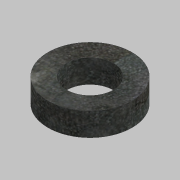
# Autodesk Inventor part: Two Piece Clamp Huco Stock No 046201030 Dim 30-54-15
Saved by Autodesk Inventor 2020.1 (Build 241239000, 239)
## iProperties
Created: 2019-08-27
Part Number: Two Piece Clamp Huco Stock No 046201030 Dim 30-54-15
Material: Steel
Document SubType Name: Modeling
Designer: Oliver Frolovs
Density: 7.85 g/cm^3
Appearance: Plate
Mass: 186.441 g
Surface Area: 71.2513 cm^2
Volume: 23.7504 cm^3
Huco30_54_15_TwoPieceClampWidth: 15.000 mm
Huco30_54_15_TwoPieceClampBore: 30.000 mm
Huco30_54_15_TwoPieceClampOuterDiameter: 54.000 mm
Author: Oliver Frolovs
Autodesk Inventor part; units mm, degrees
ref_plane "YZ Plane" through (0, 0, 0) normal (1, 0, 0) x (0, 1, 0)
ref_plane "XZ Plane" through (0, 0, 0) normal (0, 1, 0) x (-1, 0, 0)
ref_plane "XY Plane" through (0, 0, 0) normal (0, 0, 1) x (1, 0, 0)
sketch "Two Piece Clamp Profile" plane through (0, 0, 0) normal (0, 0, 1) x (1, 0, 0)
  circle A0 centre (0, 0) radius 15
  circle A1 centre (0, 0) radius 27
  dimension "d0" = 54
  dimension "d1" = 30
  constraints: 2 centre point, 2 coincident
  measures "d0" diameter of A1
  measures "d1" diameter of A0
extrude "Make Clamp by Extrusion" add sketch "Two Piece Clamp Profile" along normal mid plane 15
equation "\"d0\" = Huco30_54_15_TwoPieceClampOuterDiameter"
equation "\"d1\" = Huco30_54_15_TwoPieceClampBore"
equation "\"d2\" = Huco30_54_15_TwoPieceClampWidth"
equation "\"Huco30_54_15_TwoPieceClampWidth\" = 15"
equation "\"Huco30_54_15_TwoPieceClampBore\" = 30"
equation "\"Huco30_54_15_TwoPieceClampOuterDiameter\" = 54"
body "Solid1"
